Autodesk Fusion 360 part; units mm, degrees
(part 2 of 2)
  spline S18 degree 5 poles (-4.9086, 5.0572) (-4.9127, 5.0613) (-4.9209, 5.0695) (-4.9336, 5.0813) (-4.9513, 5.0962) (-4.9744, 5.1137) (-4.9983, 5.1304) (-5.0226, 5.1466) (-5.0472, 5.1625) (-5.072, 5.1783) (-5.097, 5.1938) (-5.1223, 5.2091) (-5.1478, 5.224) (-5.1737, 5.2385) (-5.2, 5.2525) (-5.2266, 5.2662) (-5.2535, 5.2796) (-5.2806, 5.2926) (-5.3079, 5.3054) (-5.3354, 5.318) (-5.3631, 5.3303) (-5.391, 5.3423) (-5.4191, 5.3541) (-5.4474, 5.3656) (-5.476, 5.3768) (-5.5047, 5.3878) (-5.5336, 5.3984) (-5.5627, 5.4089) (-5.592, 5.4191) (-5.6215, 5.429) (-5.6511, 5.4387) (-5.6809, 5.4482) (-5.7108, 5.4574) (-5.7409, 5.4664) (-5.7712, 5.4751) (-5.8016, 5.4836) (-5.8322, 5.4919) (-5.8629, 5.4999) (-5.8938, 5.5077) (-5.9248, 5.5153) (-5.9559, 5.5226) (-5.9872, 5.5297) (-6.0186, 5.5366) (-6.0501, 5.5433) (-6.0818, 5.5497) (-6.1136, 5.5559) (-6.1456, 5.5619) (-6.1776, 5.5676) (-6.2098, 5.5731) (-6.2421, 5.5784) (-6.2745, 5.5835) (-6.307, 5.5884) (-6.3397, 5.593) (-6.3724, 5.5975) (-6.4053, 5.6017) (-6.4383, 5.6056) (-6.4713, 5.6094) (-6.5045, 5.613) (-6.5378, 5.6163) (-6.5712, 5.6194) (-6.6046, 5.6223) (-6.6382, 5.625) (-6.6719, 5.6274) (-6.7056, 5.6297) (-6.7395, 5.6317) (-6.7734, 5.6335) (-6.8075, 5.6351) (-6.8416, 5.6365) (-6.8758, 5.6377) (-6.9101, 5.6386) (-6.9444, 5.6394) (-6.972, 5.6398) (-6.9927, 5.64) (-7.0065, 5.6401) (-7.0134, 5.6402) knots 0 0 0 0 0 0 0.01428571 0.02857143 0.04285714 0.05714286 0.07142857 0.08571429 0.1 0.11428571 0.12857143 0.14285714 0.15714286 0.17142857 0.18571429 0.2 0.21428571 0.22857143 0.24285714 0.25714286 0.27142857 0.28571429 0.3 0.31428571 0.32857143 0.34285714 0.35714286 0.37142857 0.38571429 0.4 0.41428571 0.42857143 0.44285714 0.45714286 0.47142857 0.48571429 0.5 0.51428571 0.52857143 0.54285714 0.55714286 0.57142857 0.58571429 0.6 0.61428571 0.62857143 0.64285714 0.65714286 0.67142857 0.68571429 0.7 0.71428571 0.72857143 0.74285714 0.75714286 0.77142857 0.78571429 0.8 0.81428571 0.82857143 0.84285714 0.85714286 0.87142857 0.88571429 0.9 0.91428571 0.92857143 0.94285714 0.95714286 0.97142857 0.98571429 1 1 1 1 1 1
  arc A38 (-7.0134, 5.6402) -> (-7.5314, 4.9273) centre (0, 0) ccw
  spline S19 degree 5 poles (-7.5314, 4.9273) (-7.5292, 4.9207) (-7.5249, 4.9076) (-7.5182, 4.888) (-7.5093, 4.8619) (-7.498, 4.8294) (-7.4865, 4.7971) (-7.4748, 4.765) (-7.4629, 4.7329) (-7.4509, 4.7011) (-7.4387, 4.6693) (-7.4263, 4.6378) (-7.4137, 4.6064) (-7.401, 4.5751) (-7.3881, 4.544) (-7.375, 4.5131) (-7.3617, 4.4823) (-7.3482, 4.4516) (-7.3346, 4.4212) (-7.3208, 4.3909) (-7.3068, 4.3608) (-7.2927, 4.3308) (-7.2784, 4.301) (-7.2639, 4.2714) (-7.2492, 4.242) (-7.2343, 4.2127) (-7.2193, 4.1837) (-7.2041, 4.1548) (-7.1887, 4.1261) (-7.1732, 4.0976) (-7.1574, 4.0692) (-7.1415, 4.0411) (-7.1255, 4.0131) (-7.1092, 3.9854) (-7.0928, 3.9578) (-7.0762, 3.9305) (-7.0594, 3.9033) (-7.0425, 3.8764) (-7.0253, 3.8496) (-7.008, 3.8231) (-6.9905, 3.7968) (-6.9729, 3.7707) (-6.955, 3.7449) (-6.937, 3.7192) (-6.9188, 3.6938) (-6.9004, 3.6687) (-6.8819, 3.6437) (-6.8631, 3.619) (-6.8442, 3.5946) (-6.8251, 3.5704) (-6.8058, 3.5464) (-6.7863, 3.5227) (-6.7667, 3.4994) (-6.7468, 3.4763) (-6.7267, 3.4534) (-6.7064, 3.4309) (-6.686, 3.4086) (-6.6654, 3.3866) (-6.6446, 3.3649) (-6.6236, 3.3434) (-6.6024, 3.3224) (-6.5809, 3.3017) (-6.5591, 3.2816) (-6.537, 3.2619) (-6.5147, 3.2426) (-6.4922, 3.2236) (-6.4695, 3.2049) (-6.4468, 3.1864) (-6.4239, 3.1683) (-6.4006, 3.1507) (-6.3768, 3.1341) (-6.3572, 3.1219) (-6.342, 3.1135) (-6.3317, 3.1082) (-6.3265, 3.1056) knots -1 -1 -1 -1 -1 -1 -0.98571429 -0.97142857 -0.95714286 -0.94285714 -0.92857143 -0.91428571 -0.9 -0.88571429 -0.87142857 -0.85714286 -0.84285714 -0.82857143 -0.81428571 -0.8 -0.78571429 -0.77142857 -0.75714286 -0.74285714 -0.72857143 -0.71428571 -0.7 -0.68571429 -0.67142857 -0.65714286 -0.64285714 -0.62857143 -0.61428571 -0.6 -0.58571429 -0.57142857 -0.55714286 -0.54285714 -0.52857143 -0.51428571 -0.5 -0.48571429 -0.47142857 -0.45714286 -0.44285714 -0.42857143 -0.41428571 -0.4 -0.38571429 -0.37142857 -0.35714286 -0.34285714 -0.32857143 -0.31428571 -0.3 -0.28571429 -0.27142857 -0.25714286 -0.24285714 -0.22857143 -0.21428571 -0.2 -0.18571429 -0.17142857 -0.15714286 -0.14285714 -0.12857143 -0.11428571 -0.1 -0.08571429 -0.07142857 -0.05714286 -0.04285714 -0.02857143 -0.01428571 0 0 0 0 0 0
  line L19 (-6.3265, 3.1056) -> (-5.744, 2.8188)
  arc A39 (-5.341, 1.8404) -> (-5.744, 2.8188) centre (-6.0973, 2.1011) ccw
  circle A40 centre (0, 0) radius 2.7552
component "Spur Gear (10 teeth)" placed x (1, 0, 0) y (0, 1, 0) z (0, 0, 1) at (0, 0, 0)
equation "teethnum = 20"
